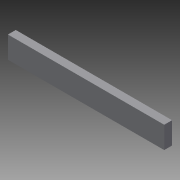
# Autodesk Inventor part: 知能ロボコン砲台スペーサ高さ
Saved by Autodesk Inventor 2013 (Build 170138000, 138)
## iProperties
Created: 2014-07-01
Part Number: 知能ロボコン砲台スペーサ高さ
Material: 一般
Document SubType Name: Modeling
Designer: horumo136
Density: 1 g/cm^3
Author: horumo136
Autodesk Inventor part; units mm, degrees
ref_plane "YZ Plane" through (0, 0, 0) normal (1, 0, 0) x (0, 1, 0)
ref_plane "XZ Plane" through (0, 0, 0) normal (0, 1, 0) x (-1, 0, 0)
ref_plane "XY Plane" through (0, 0, 0) normal (0, 0, 1) x (1, 0, 0)
sketch "スケッチ1" plane through (0, 0, 0) normal (0, 1, 0) x (-1, 0, 0)
  line L0 (0, 0) -> (-90, 0)
  line L1 (-90, 0) -> (-90, 10)
  line L2 (-90, 10) -> (0, 10)
  line L3 (0, 10) -> (0, 0)
  dimension "d0" = 90
  dimension "d1" = 10
  constraints: 8 end point, 2 parallel, 1 horizontal, 1 perpendicular
  measures "d0" distance of L1.end L2.end
  measures "d1" distance of L0.end L1.end
extrude "押し出し1" add sketch "スケッチ1" along normal blind 0.5
sketch "スケッチ2" plane through (0, 0, 0) normal (-1, 0, 0) x (0, 0, 1)
  line L0 (10, 0) -> (0, 0) projected
  line L1 (10, 0) -> (10, 0.5) projected
  line L2 (0, 0.5) -> (10, 0.5) projected
  line L3 (0, 0) -> (0, 0.5) projected
  line L4 (0, 0) -> (10, 0)
  line L5 (10, 0) -> (10, 5)
  line L6 (10, 5) -> (0, 5)
  line L7 (0, 5) -> (0, 0)
  dimension "d4" = 5
  constraints: 8 end point, 2 parallel, 1 horizontal, 1 perpendicular
  measures "d4" distance of L5.end L4.end
extrude "押し出し2" add sketch "スケッチ2" along normal blind 5 contours L2 L7 L6 L5
sketch "スケッチ3" plane through (0, 0, 0) normal (-1, 0, 0) x (0, 0, 1)
  line L0 (10, 0) -> (0, 0) projected
  line L1 (10, 0) -> (10, 0.5) projected
  line L2 (0, 0.5) -> (10, 0.5) projected
  line L3 (0, 0) -> (0, 0.5) projected
extrude "押し出し3" add sketch "スケッチ3" along normal blind 5
sketch "スケッチ4" plane through (90, 0, 10) normal (1, 0, 0) x (0, 0, -1)
  line L0 (0, 0) -> (10, 0)
  line L1 (10, 0) -> (10, 5.0408)
  line L2 (10, 5.0408) -> (0, 5.0408)
  line L3 (0, 5.0408) -> (0, 0)
  constraints: 8 end point, 2 parallel, 1 horizontal, 1 perpendicular
extrude "押し出し4" add sketch "スケッチ4" along normal blind 5
sketch "スケッチ5" plane through (0, 0.5, 0) normal (0, 0, -1) x (-1, 0, 0)
  line L0 (5, -0.5) -> (-95, -0.5) projected
  line L1 (5, 4.5) -> (5, -0.5) projected
  line L2 (0, 4.5) -> (5, 4.5) projected
  line L3 (0, 4.5) -> (0, 0) projected
  line L4 (-90, 0) -> (0, 0) projected
  line L5 (-90, 0) -> (-90, 4.5408) projected
  line L6 (-90, 4.5408) -> (-95, 4.5408) projected
  line L7 (-95, -0.5) -> (-95, 4.5408) projected
  line L8 (-95, -0.5) -> (5, -0.5)
  line L9 (5, -0.5) -> (5, 4.5)
  line L10 (5, 4.5) -> (-95, 4.5)
  line L11 (-95, 4.5) -> (-95, -0.5)
  point P0 (0, -0.5)
  constraints: 8 end point, 2 parallel, 1 horizontal, 1 perpendicular
extrude "押し出し5" add sketch "スケッチ5" along normal blind 2
sketch "スケッチ6" plane through (0, 0.5, 10) normal (0, 0, 1) x (1, 0, 0)
  line L0 (95, -0.5) -> (-5, -0.5) projected
  line L1 (95, 4.5408) -> (95, -0.5) projected
  line L2 (-5, -0.5) -> (95, -0.5)
  line L3 (95, -0.5) -> (95, 4.5408)
  line L4 (95, 4.5408) -> (-5, 4.5408)
  line L5 (-5, 4.5408) -> (-5, -0.5)
  point P0 (0, -0.5)
  constraints: 8 end point, 2 parallel, 1 horizontal, 1 perpendicular
extrude "押し出し6" add sketch "スケッチ6" along normal blind 2
